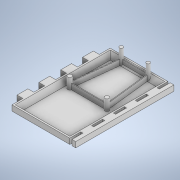
# Autodesk Inventor part: rfid_top
Saved by Autodesk Inventor 2020 (Build 240168000, 168)
## iProperties
Created: 2019-06-30
Part Number: rfid_top
Material: Generic
Document SubType Name: Modeling
Designer: jjsch
Density: 1 g/cm^3
Appearance: Default
Author: jjsch
Autodesk Inventor part; units mm, degrees
ref_plane "YZ Plane" through (0, 0, 0) normal (1, 0, 0) x (0, 1, 0)
ref_plane "XZ Plane" through (0, 0, 0) normal (0, 1, 0) x (-1, 0, 0)
ref_plane "XY Plane" through (0, 0, 0) normal (0, 0, 1) x (1, 0, 0)
sketch "Sketch1" plane through (0, 0, 0) normal (0, 1, 0) x (-1, 0, 0)
  line L0 (-31.9185, 45) -> (31.9185, 45)
  line L1 (31.9185, 45) -> (31.9185, -45)
  line L2 (31.9185, -45) -> (-31.9185, -45)
  line L3 (-31.9185, -45) -> (-31.9185, 45)
  line L4 (-31.9185, 45) -> (31.9185, -45) construction
  line L5 (31.9185, 45) -> (-31.9185, -45) construction
  point P0 (0, 0)
  dimension "d0" = 63.837
  dimension "d1" = 90
  constraints: 12 end point, 2 midpoint, 2 parallel, 1 horizontal, 1 perpendicular
  measures "d0" distance of L1.end L2.end
  measures "d1" distance of L0.end L1.end
extrude "Extrusion1" add sketch "Sketch1" along normal blind 5
sketch "Sketch2" plane through (0, 5, 0) normal (0, 1, 0) x (1, 0, 0)
  line L0 (31.9185, -45) -> (31.9185, 45) projected
  line L1 (31.9185, -45) -> (26.4995, -45)
  line L2 (26.4995, -45) -> (26.4995, -35)
  line L3 (26.4995, -35) -> (31.9185, -35)
  line L4 (31.9185, -35) -> (31.9185, -45)
  line L5 (-31.9185, 45) -> (-31.9185, -45) projected
  line L6 (-31.9185, -45) -> (-26.4995, -45)
  line L7 (-26.4995, -45) -> (-26.4995, -35)
  line L8 (-26.4995, -35) -> (-31.9185, -35)
  line L9 (-31.9185, -35) -> (-31.9185, -45)
  line L10 (31.9185, -25) -> (26.4995, -25)
  line L11 (26.4995, -25) -> (26.4995, -15)
  line L12 (26.4995, -15) -> (31.9185, -15)
  line L13 (31.9185, -15) -> (31.9185, -25)
  line L14 (-31.9185, -25) -> (-26.4995, -25)
  line L15 (-26.4995, -25) -> (-26.4995, -15)
  line L16 (-26.4995, -15) -> (-31.9185, -15)
  line L17 (-31.9185, -15) -> (-31.9185, -25)
  line L18 (31.9185, -5) -> (26.4995, -5)
  line L19 (26.4995, -5) -> (26.4995, 5)
  line L20 (26.4995, 5) -> (31.9185, 5)
  line L21 (31.9185, 5) -> (31.9185, -5)
  line L22 (-31.9185, -5) -> (-26.4995, -5)
  line L23 (-26.4995, -5) -> (-26.4995, 5)
  line L24 (-26.4995, 5) -> (-31.9185, 5)
  line L25 (-31.9185, 5) -> (-31.9185, -5)
  line L26 (31.9185, 15) -> (26.4995, 15)
  line L27 (26.4995, 15) -> (26.4995, 25)
  line L28 (26.4995, 25) -> (31.9185, 25)
  line L29 (31.9185, 25) -> (31.9185, 15)
  line L30 (-31.9185, 15) -> (-26.4995, 15)
  line L31 (-26.4995, 15) -> (-26.4995, 25)
  line L32 (-26.4995, 25) -> (-31.9185, 25)
  line L33 (-31.9185, 25) -> (-31.9185, 15)
  line L34 (31.9185, 35) -> (26.4995, 35)
  line L35 (26.4995, 35) -> (26.4995, 45)
  line L36 (26.4995, 45) -> (31.9185, 45)
  line L37 (31.9185, 45) -> (31.9185, 35)
  line L38 (-31.9185, 35) -> (-26.4995, 35)
  line L39 (-26.4995, 35) -> (-26.4995, 45)
  line L40 (-26.4995, 45) -> (-31.9185, 45)
  line L41 (-31.9185, 45) -> (-31.9185, 35)
  point P0 (0, 0)
  dimension "d4" = 5.419
  dimension "d5" = 10
  dimension "d6" = 5.419
  dimension "d7" = 10
  dimension "d10" = 20
  constraints: 80 end point, 4 parallel, 2 horizontal, 2 perpendicular, 1 vertical, 64 other
  measures "d4" distance of L2.end L3.end
  measures "d5" distance of L1.end L2.end
  measures "d6" distance of L8.end L7.end
  measures "d7" distance of L7.end L6.end
  measures "d10" distance of L2.end L11.end
extrude "Extrusion2" cut sketch "Sketch2" against normal blind 5
sketch "Sketch3" plane through (0, 5, 0) normal (0, 1, 0) x (1, 0, 0)
  line L0 (28.4995, -45) -> (31.9185, -45)
  line L1 (31.9185, -45) -> (31.9185, 45)
  line L2 (31.9185, 45) -> (28.4995, 45)
  line L3 (28.4995, 45) -> (28.4995, -45)
  line L4 (-26.4995, -45) -> (26.4995, -45) projected
  line L5 (26.4995, -45) -> (26.4995, -35) projected
  point P0 (0, 0)
  dimension "d17" = 90
  dimension "d18" = 3.419
  dimension "d19" = 0
  dimension "d20" = 2
  constraints: 8 end point, 2 parallel, 1 horizontal, 1 perpendicular
  measures "d17" distance of L1.end L0.end
  measures "d18" distance of L0.start L0.end
  measures "d19" distance between parallel lines of L4 L0
  measures "d20" distance between parallel lines of L5 L3
extrude "Extrusion3" add sketch "Sketch3" against normal blind 5
sketch "Sketch4" plane through (0, 5, 0) normal (0, 1, 0) x (1, 0, 0)
  line L0 (31.9185, -45) -> (31.9185, 45) projected
  line L1 (31.9185, 45) -> (28.4995, 45) projected
  line L2 (28.4995, 45) -> (28.4995, 35) projected
  line L3 (28.4995, 35) -> (26.4995, 35) projected
  line L4 (26.4995, 35) -> (26.4995, 45) projected
  line L5 (26.4995, 45) -> (-26.4995, 45) projected
  line L6 (-26.4995, 45) -> (-26.4995, 35) projected
  line L7 (-26.4995, 35) -> (-31.9185, 35) projected
  line L8 (-31.9185, 35) -> (-31.9185, 25) projected
  line L9 (-31.9185, 25) -> (-26.4995, 25) projected
  line L10 (-26.4995, 25) -> (-26.4995, 15) projected
  line L11 (-26.4995, 15) -> (-31.9185, 15) projected
  line L12 (-31.9185, 15) -> (-31.9185, 5) projected
  line L13 (-31.9185, 5) -> (-26.4995, 5) projected
  line L14 (-26.4995, 5) -> (-26.4995, -5) projected
  line L15 (-26.4995, -5) -> (-31.9185, -5) projected
  line L16 (-31.9185, -5) -> (-31.9185, -15) projected
  line L17 (-31.9185, -15) -> (-26.4995, -15) projected
  line L18 (-26.4995, -15) -> (-26.4995, -25) projected
  line L19 (-26.4995, -25) -> (-31.9185, -25) projected
  line L20 (-31.9185, -25) -> (-31.9185, -35) projected
  line L21 (-31.9185, -35) -> (-26.4995, -35) projected
  line L22 (-26.4995, -35) -> (-26.4995, -45) projected
  line L23 (-26.4995, -45) -> (26.4995, -45) projected
  line L24 (26.4995, -45) -> (26.4995, -35) projected
  line L25 (26.4995, -35) -> (28.4995, -35) projected
  line L26 (28.4995, -35) -> (28.4995, -45) projected
  line L27 (28.4995, -45) -> (31.9185, -45) projected
  line L28 (28.4995, 25) -> (28.4995, 15) projected
  line L29 (28.4995, 15) -> (26.4995, 15) projected
  line L30 (26.4995, 15) -> (26.4995, 25) projected
  line L31 (26.4995, 25) -> (28.4995, 25) projected
  line L32 (28.4995, 5) -> (28.4995, -5) projected
  line L33 (28.4995, -5) -> (26.4995, -5) projected
  line L34 (26.4995, -5) -> (26.4995, 5) projected
  line L35 (26.4995, 5) -> (28.4995, 5) projected
  line L36 (28.4995, -15) -> (28.4995, -25) projected
  line L37 (28.4995, -25) -> (26.4995, -25) projected
  line L38 (26.4995, -25) -> (26.4995, -15) projected
  line L39 (26.4995, -15) -> (28.4995, -15) projected
  line L40 (-20.9995, 39.5) -> (20.9995, 39.5)
  line L41 (20.9995, 39.5) -> (20.9995, 29.5)
  line L42 (20.9995, 29.5) -> (26.4185, 29.5)
  line L43 (26.4185, 29.5) -> (26.4185, -29.5)
  line L44 (26.4185, -29.5) -> (20.9995, -29.5)
  line L45 (20.9995, -29.5) -> (20.9995, -39.5)
  line L46 (20.9995, -39.5) -> (-20.9995, -39.5)
  line L47 (-20.9995, -39.5) -> (-20.9995, -30.5)
  line L48 (-20.9995, -30.5) -> (-20.9995, -10.5)
  line L49 (-20.9995, -10.5) -> (-20.9995, 9.5)
  line L50 (-20.9995, 9.5) -> (-20.9995, 29.5)
  line L51 (-20.9995, 29.5) -> (-20.9995, 39.5)
  line L52 (20.9995, 29.5) -> (20.9995, -29.5)
  point P0 (0, 0)
  dimension "d23" = 5.5
  constraints: 26 end point, 1 collinear, 11 other
  measures "d23" distance between parallel lines of L5 L40
extrude "Extrusion4" cut sketch "Sketch4" against normal blind 4 contours L40 L41 L52 L45 L46 L47 L48 L49 L50 L51
chamfer "Chamfer1" distance 4 angle 45 4 edges at (-20.9995, 5, 0) (0, 5, -39.5) (20.9995, 5, 0) (0, 5, 39.5)
sketch "Sketch5" plane through (0, 0, 0) normal (0, -1, 0) x (1, 0, 0)
  circle A0 centre (-12.35, -41) radius 1.6
  circle A1 centre (12.35, -41) radius 1.6
  circle A2 centre (-17.05, 1.5) radius 1.9
  circle A3 centre (17.05, 1.5) radius 1.9
  line L0 (-26.4995, 45) -> (26.4995, 45) projected
  line L1 (26.4995, -45) -> (-26.4995, -45) projected
  point P0 (0, 0)
  dimension "d29" = 3.2
  dimension "d30" = 3.2
  dimension "d31" = 24.7
  dimension "d32" = 12.35
  dimension "d33" = 3.8
  dimension "d34" = 3.8
  dimension "d37" = 42.5
  dimension "d39" = 4.7
  dimension "d40" = 4.7
  dimension "d41" = 43.5
  dimension "d42" = 4
  constraints: 4 centre point, 2 horizontal alignment
  measures "d29" diameter of A0
  measures "d30" diameter of A1
  measures "d31" distance of A1.centre A0.centre
  measures "d32" horizontal distance of point (0, 0) A1.centre
  measures "d33" diameter of A2
  measures "d34" diameter of A3
  measures "d37" vertical distance of A0.centre A2.centre
  measures "d39" horizontal distance of A2.centre A0.centre
  measures "d40" horizontal distance of A3.centre A1.centre
  measures "d41" distance from line of L0 A2.centre
  measures "d42" distance from line of L1 A0.centre
extrude "Extrusion5" add sketch "Sketch5" against normal blind 15
sketch "Sketch6" plane through (0, 1, 0) normal (0, 1, 0) x (1, 0, 0)
  circle A0 centre (17.05, -1.5) radius 1.9 projected
  circle A1 centre (-17.05, -1.5) radius 1.9 projected
  circle A2 centre (-12.35, 41) radius 1.6 projected
  circle A3 centre (12.35, 41) radius 1.6 projected
  line L0 (17.05, -1.5) -> (-17.05, -1.5)
  arc A4 (12.9068, 39.5) -> (11.7932, 39.5) centre (12.35, 41) ccw projected
  line L1 (17.05, -1.5) -> (12.35, 41)
  line L2 (12.35, 41) -> (-12.35, 41)
  line L3 (-12.35, 41) -> (-17.05, -1.5)
  arc A5 (-11.7932, 39.5) -> (-12.9068, 39.5) centre (-12.35, 41) ccw projected
  line L4 (-12.35, 41) -> (12.35, 41)
  line L5 (12.3887, 41.35) -> (-12.3887, 41.35)
  line L6 (-12.3887, 41.35) -> (-12.3887, 40.65)
  line L7 (-12.3887, 40.65) -> (12.3887, 40.65)
  line L8 (12.3887, 40.65) -> (12.3887, 41.35)
  line L9 (12.3887, 41.35) -> (-12.3887, 40.65) construction
  line L10 (-12.3887, 41.35) -> (12.3887, 40.65) construction
  line L11 (-12.0021, 40.9615) -> (-16.7021, -1.5385)
  line L12 (-16.7021, -1.5385) -> (-17.3979, -1.4615)
  line L13 (-17.3979, -1.4615) -> (-12.6979, 41.0385)
  line L14 (-12.6979, 41.0385) -> (-12.0021, 40.9615)
  line L15 (-12.0021, 40.9615) -> (-17.3979, -1.4615) construction
  line L16 (-16.7021, -1.5385) -> (-12.6979, 41.0385) construction
  line L17 (-17.05, -1.15) -> (17.05, -1.15)
  line L18 (17.05, -1.15) -> (17.05, -1.85)
  line L19 (17.05, -1.85) -> (-17.05, -1.85)
  line L20 (-17.05, -1.85) -> (-17.05, -1.15)
  line L21 (-17.05, -1.15) -> (17.05, -1.85) construction
  line L22 (17.05, -1.15) -> (-17.05, -1.85) construction
  line L23 (17.4356, -1.8031) -> (12.6601, 41.38)
  line L24 (12.6601, 41.38) -> (11.9644, 41.3031)
  line L25 (11.9644, 41.3031) -> (16.7399, -1.88)
  line L26 (16.7399, -1.88) -> (17.4356, -1.8031)
  line L27 (17.4356, -1.8031) -> (11.9644, 41.3031) construction
  line L28 (12.6601, 41.38) -> (16.7399, -1.88) construction
  point P0 (0, 0)
  point P1 (0, 41)
  point P2 (-14.7, 19.75)
  point P3 (0, -1.5)
  point P4 (14.7, 19.75)
  point P5 (-12.3887, 41.0043)
  point P6 (-17.05, -1.5)
  point P7 (16.7366, -1.85)
  point P8 (17.0113, -1.85)
  point P9 (17.05, -1.8457)
  point P10 (-12.0366, 40.65)
  point P11 (12.0366, 40.65)
  point P12 (16.6592, -1.15)
  point P13 (-16.6592, -1.15)
  dimension "d45" = 0.7
  dimension "d46" = 0.7
  dimension "d47" = 0.7
  dimension "d48" = 0.7
  constraints: 58 end point, 12 midpoint, 10 parallel, 4 horizontal, 4 perpendicular, 1 collinear, 1 point on line
  measures "d45" distance of L6.end L5.end
  measures "d46" distance of L11.end L12.end
  measures "d47" distance of L17.end L18.end
  measures "d48" distance of L24.end L23.end
extrude "Extrusion6" add sketch "Sketch6" along normal blind 5 contours L23 L26 L18 L17 L1 A0 | A0 L1 A3 L23 | L19 A1 L0 A0 | A0 L0 L25 L19 | L1 L17 L25 A0 | A0 L25 A3 L1 | A3 L1 L8 L24 L23 | L0 A1 L17 A0 | A0 L17 L25 L0 | L25 L0 L18 L26 L19 | L19 L26 L25 | L19 L20 L12 L11 L0 A1 | L17 L18 L1 | L1 L0 L25 L17 | A3 L25 L7 L1 | L18 L19 L26 | L0 L11 L17 A1 | L13 A2 L3 A1 | A1 L3 L17 L20 L12 L13 | L7 L25 L2 L1 | L1 L2 L25 L24 L8 | L24 L25 L2 A3 L5 | L11 L12 L0 | L0 L3 L17 L11 | L3 A2 L11 A1 | A1 L11 L17 L3 | L13 L14 L6 L3 A2 | L20 L17 L3 | L7 A3 L2 L25 | A3 L2 A2 L5 | L3 L7 L11 A2 | L7 A2 L2 A3 | A2 L2 L14 L6 L5 | L6 L14 L3 | L3 L14 L11 L7 | L7 L11 L14 L2 A2
sketch "Sketch7" plane through (17.05, 15, 1.5) normal (0, 1, 0) x (1, 0, 0)
  circle A0 centre (-34.1, 0) radius 1.9 projected
  circle A1 centre (0, 0) radius 1.9 projected
  point P0 (-17.05, 1.5)
extrude "Extrusion7" cut sketch "Sketch7" against normal blind 4
body "Solid1"
